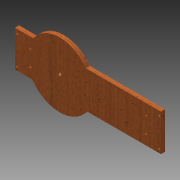
# Autodesk Inventor part: tiltStructureCrossBeam
Saved by Autodesk Inventor 2013 (Build 170138000, 138)
## iProperties
Created: 2014-06-14
Part Number: tiltStructureCrossBeam
Material: Wood (Cherry)
Document SubType Name: Modeling
Designer: Byron
Density: 0.5 g/cm^3
Mass: 49.6326 g
Surface Area: 357.646 cm^2
Volume: 99.2651 cm^3
Author: Byron
Autodesk Inventor part; units mm, degrees
ref_plane "YZ Plane" through (0, 0, 0) normal (1, 0, 0) x (0, 1, 0)
ref_plane "XZ Plane" through (0, 0, 0) normal (0, 1, 0) x (-1, 0, 0)
ref_plane "XY Plane" through (0, 0, 0) normal (0, 0, 1) x (1, 0, 0)
sketch "Sketch1" plane through (0, 0, 0) normal (0, 0, 1) x (1, 0, 0)
  line L0 (0, 78.0122) -> (0, 82.508) projected
  line L1 (-6.35, 82.508) -> (-6.35, 78.0122) projected
  line L2 (-6.35, 78.0122) -> (0, 78.0122) projected
  line L3 (222.25, 130.6664) -> (222.25, 135.1622) projected
  line L4 (215.9, 135.1622) -> (222.25, 135.1622) projected
  line L5 (215.9, 135.1622) -> (215.9, 130.6664) projected
  line L6 (222.25, 77.5379) -> (222.25, 135.1622)
  line L7 (-6.35, 134.6915) -> (-6.35, 78.0122)
  arc A0 (65.1726, 108.6235) -> (63.7223, 104.0872) centre (63.7223, 106.5872) ccw projected
  line L8 (222.25, 135.1622) -> (104.7076, 135.1622)
  line L9 (22.4128, 134.6915) -> (-6.35, 134.6915)
  line L10 (-6.35, 78.0122) -> (20.7049, 78.0122)
  line L11 (106.4207, 77.5379) -> (222.25, 77.5379)
  arc A1 (104.7076, 135.1622) -> (22.4128, 134.6915) centre (63.7223, 106.5872) ccw
  arc A2 (20.7049, 78.0122) -> (106.4207, 77.5379) centre (63.7223, 106.5872) ccw
  line L12 (215.9, 130.6664) -> (222.25, 130.6664) projected
  line L13 (0, 82.508) -> (-6.35, 82.508) projected
  point P0 (0, 0)
  constraints: 12 end point, 5 parallel, 4 point on circle, 2 centre point, 2 horizontal, 2 perpendicular, 1 coincident
extrude "Extrusion1" add sketch "Sketch1" along normal blind 6.35
sketch "Sketch2" plane through (0, 0, 0) normal (0, 0, -1) x (-1, 0, 0)
  line L0 (-53.2456, 114.8496) -> (-74.1989, 114.8496) projected
  line L1 (-13.716, 122.4622) -> (-13.716, 90.7122) projected
  line L2 (-63.7223, 114.8496) -> (-63.7223, 83.3208) construction
  line L3 (-13.716, 106.5872) -> (-74.4954, 106.5872) construction
  arc A0 (-63.7223, 109.0872) -> (-61.2223, 106.5872) centre (-63.7223, 106.5872) ccw
  line L4 (-63.7223, 109.0872) -> (-62.2719, 104.5509)
  point P0 (0, 0)
  dimension "d2" = 5
  dimension "d3" = 4.7625
  constraints: 6 end point, 4 point on line, 3 point on circle, 2 midpoint, 1 centre point, 1 parallel, 1 perpendicular
  measures "d2" diameter of A0
  measures "d3" distance of L4.start L4.end
extrude "Extrusion2" cut sketch "Sketch2" against normal through all
sketch "Sketch3" plane through (0, 0, 0) normal (0, 0, -1) x (-1, 0, 0)
  line L0 (6.35, 134.6915) -> (6.35, 78.0122) construction
  line L1 (-222.25, 135.1622) -> (-104.7076, 135.1622) construction
  line L2 (-222.25, 77.5379) -> (-222.25, 135.1622) construction
  line L3 (-106.4207, 77.5379) -> (-222.25, 77.5379) construction
  line L4 (-215.9, 135.1622) -> (-215.9, 130.6664) construction
  line L5 (-217.6131, 96.5879) -> (-200.4173, 96.5879) construction
  line L6 (-200.4173, 90.2379) -> (-217.6131, 90.2379) construction
  line L7 (-217.6131, 90.2379) -> (-217.6131, 96.5879) construction
  line L8 (-217.6131, 121.9879) -> (-200.4173, 121.9879) construction
  line L9 (-200.4173, 115.6379) -> (-217.6131, 115.6379) construction
  line L10 (-217.6131, 115.6379) -> (-217.6131, 121.9879) construction
  circle A0 centre (-219.075, 128.8122) radius 1.8542
  circle A1 centre (-198.5631, 118.8129) radius 1.8542
  line L11 (-222.25, 106.3501) -> (-215.9, 106.3501) construction
  circle A2 centre (-219.075, 83.8879) radius 1.8542
  circle A3 centre (-198.5631, 93.8872) radius 1.8542
  line L12 (-107.95, 135.1622) -> (-107.95, 78.0122) construction
  circle A4 centre (3.175, 128.8122) radius 1.8542
  circle A5 centre (-17.3369, 118.8129) radius 1.8542
  circle A6 centre (-17.3369, 93.8872) radius 1.8542
  circle A7 centre (3.175, 83.8879) radius 1.8542
  line L13 (-200.4173, 121.9879) -> (-200.4173, 115.6379) projected
  line L14 (-200.4173, 96.5879) -> (-200.4173, 90.2379) projected
  point P0 (0, 0)
  point P1 (-215.9, 135.1622)
  dimension "d7" = 3.7084
  dimension "d8" = 3.175
  dimension "d9" = 3.175
  dimension "d10" = 6.35
  dimension "d11" = 3.7084
  dimension "d12" = 19.05
  dimension "d13" = 28.8121
  dimension "d14" = 28.8121
  dimension "d15" = 114.3
  dimension "d16" = 114.3
  constraints: 8 centre point, 6 symmetric about line, 4 end point, 8 other
  measures "d7" diameter of A0
  measures "d8" distance from line of A0.centre L2
  measures "d10" distance from line of A0.centre L1
  measures "d11" diameter of A1
  measures "d12" distance from line of L10 A1.centre
  measures "d14" distance between parallel lines of L1 L11
  measures "d15" distance between parallel lines of L2 L12
  measures "d16" distance between parallel lines of L0 L12
extrude "Extrusion3" cut sketch "Sketch3" against normal through all
equation "\"d8\" = d9"
equation "\"d13\" = d14"
equation "\"d15\" = d16"
body "Solid1"
